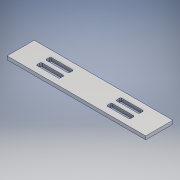
# Autodesk Inventor part: BK-BKT120-Front
Saved by Autodesk Inventor 2017 (Build 210142000, 142)
## iProperties
Created: 2016-09-24
Part Number: BK-BKT120-Front
Material: Aluminum 6061
Document SubType Name: Modeling
Designer: vslabsal
Density: 2.7 g/cm^3
Appearance: Aluminum - Flat
Author: vslabsal
Autodesk Inventor part; units mm, degrees
ref_plane "YZ Plane" through (0, 0, 0) normal (1, 0, 0) x (0, 1, 0)
ref_plane "XZ Plane" through (0, 0, 0) normal (0, 1, 0) x (-1, 0, 0)
ref_plane "XY Plane" through (0, 0, 0) normal (0, 0, 1) x (1, 0, 0)
sketch "Sketch1" plane through (0, 0, 0) normal (0, 0, 1) x (1, 0, 0)
  line L0 (-194.31, -38.1) -> (194.31, -38.1)
  line L1 (194.31, -38.1) -> (194.31, 38.1)
  line L2 (194.31, 38.1) -> (-194.31, 38.1)
  line L3 (-194.31, 38.1) -> (-194.31, -38.1)
  line L4 (-194.31, -38.1) -> (194.31, 38.1) construction
  line L5 (194.31, -38.1) -> (-194.31, 38.1) construction
  line L6 (66, 20) -> (131, 6) construction
  line L7 (131, 20) -> (66, 6) construction
  arc A0 (69.175, 20) -> (66, 16.825) centre (69.175, 16.825) ccw
  arc A1 (66, 9.175) -> (69.175, 6) centre (69.175, 9.175) ccw
  arc A2 (127.825, 6) -> (131, 9.175) centre (127.825, 9.175) ccw
  arc A3 (131, 16.825) -> (127.825, 20) centre (127.825, 16.825) ccw
  line L8 (66, 16.825) -> (66, 9.175)
  line L9 (69.175, 6) -> (127.825, 6)
  line L10 (131, 9.175) -> (131, 16.825)
  line L11 (69.175, 20) -> (127.825, 20)
  line L12 (-131, -6) -> (-66, -20) construction
  line L13 (-66, -6) -> (-131, -20) construction
  arc A4 (-127.825, -6) -> (-131, -9.175) centre (-127.825, -9.175) ccw
  arc A5 (-131, -16.825) -> (-127.825, -20) centre (-127.825, -16.825) ccw
  arc A6 (-69.175, -20) -> (-66, -16.825) centre (-69.175, -16.825) ccw
  arc A7 (-66, -9.175) -> (-69.175, -6) centre (-69.175, -9.175) ccw
  line L14 (-131, -9.175) -> (-131, -16.825)
  line L15 (-127.825, -20) -> (-69.175, -20)
  line L16 (-66, -16.825) -> (-66, -9.175)
  line L17 (-127.825, -6) -> (-69.175, -6)
  arc A8 (-66, 16.825) -> (-69.175, 20) centre (-69.175, 16.825) ccw
  line L18 (-127.825, 20) -> (-69.175, 20)
  line L19 (-127.825, 6) -> (-69.175, 6)
  line L20 (-131, 20) -> (-66, 6) construction
  line L21 (-66, 20) -> (-131, 6) construction
  line L22 (-131, 16.825) -> (-131, 9.175)
  arc A9 (-127.825, 20) -> (-131, 16.825) centre (-127.825, 16.825) ccw
  arc A10 (-131, 9.175) -> (-127.825, 6) centre (-127.825, 9.175) ccw
  line L23 (-66, 9.175) -> (-66, 16.825)
  arc A11 (-69.175, 6) -> (-66, 9.175) centre (-69.175, 9.175) ccw
  arc A12 (131, -9.175) -> (127.825, -6) centre (127.825, -9.175) ccw
  line L24 (69.175, -6) -> (127.825, -6)
  line L25 (69.175, -20) -> (127.825, -20)
  line L26 (66, -6) -> (131, -20) construction
  line L27 (131, -6) -> (66, -20) construction
  line L28 (66, -9.175) -> (66, -16.825)
  arc A13 (69.175, -6) -> (66, -9.175) centre (69.175, -9.175) ccw
  arc A14 (66, -16.825) -> (69.175, -20) centre (69.175, -16.825) ccw
  line L29 (131, -16.825) -> (131, -9.175)
  arc A15 (127.825, -20) -> (131, -16.825) centre (127.825, -16.825) ccw
  point P0 (0, 0)
  point P1 (0, 0)
  point P2 (98.5, 13)
  point P3 (-98.5, -13)
  point P4 (-98.5, 13)
  point P5 (98.5, -13)
  dimension "d0" = 388.62
  dimension "d1" = 76.2
  constraints: 60 end point, 40 point on circle, 16 centre point, 12 point on line, 10 midpoint, 9 horizontal, 8 vertical, 2 parallel, 1 perpendicular
  measures "d0" distance of L0.start L0.end
  measures "d1" distance of L0.end L1.end
extrude "Extrusion4" add sketch "Sketch1" along normal blind 9.525
body "Solid4"
